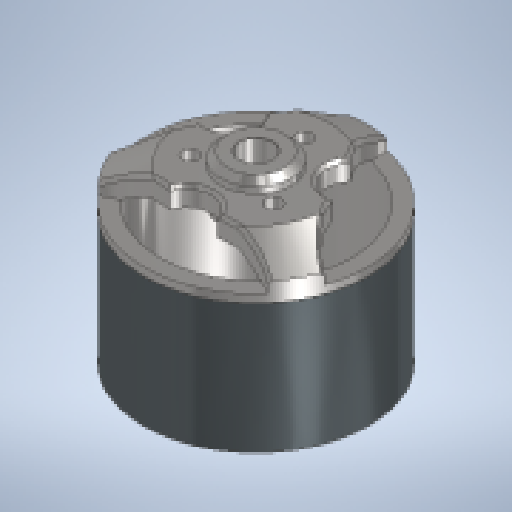
# Autodesk Inventor part: Can
Saved by Autodesk Inventor 2023.2 (Build 272271000, 271)
## iProperties
Created: 2023-03-04
Part Number: Can
Material: Stainless Steel
Document SubType Name: Modeling
Designer: Nathan Cai
Density: 8 g/cm^3
Appearance: Semi-Polished
Author: Nathan Cai
Autodesk Inventor part; units mm, degrees
ref_plane "YZ Plane" through (0, 0, 0) normal (1, 0, 0) x (0, 1, 0)
ref_plane "XZ Plane" through (0, 0, 0) normal (0, 1, 0) x (-1, 0, 0)
ref_plane "XY Plane" through (0, 0, 0) normal (0, 0, 1) x (1, 0, 0)
sketch "Sketch1" plane through (0, 0, 0) normal (0, 1, 0) x (-1, 0, 0)
  line L0 (0, 0) -> (26.5, 0)
  line L1 (26.5, 0) -> (26.5, -17.5)
  line L2 (26.5, -17.5) -> (0, -17.5)
  line L3 (0, -17.5) -> (0, 0)
  line L4 (26.5, -15) -> (0, -15)
  line L5 (0, 0) -> (21.25, 0)
  line L6 (21.25, 0) -> (21.25, -17.5)
  line L7 (21.25, -17.5) -> (0, -17.5)
  line L8 (0, -17.5) -> (0, 0)
  line L9 (26.5, 0) -> (28.5, 0)
  line L10 (28.5, 0) -> (28.5, -5.5)
  line L11 (28.5, -5.5) -> (26.5, -5.5)
  line L12 (26.5, -5.5) -> (26.5, 0)
  line L13 (28.5, 0) -> (0, 0)
  line L14 (0, 0) -> (0, -2.5)
  line L15 (0, -2.5) -> (28.5, -2.5)
  line L16 (28.5, -2.5) -> (28.5, 0)
  line L17 (26.5, -11.5) -> (23.25, -17.5)
  line L18 (26.5, -11.5) -> (23.5, -11.5) construction
  line L19 (23.5, -11.5) -> (23.5, 0)
  line L20 (23.5, 0) -> (26.5, 0)
  line L21 (26.5, 0) -> (26.5, -11.5)
  line L22 (23.5, -11.5) -> (21.6042, -15)
  line L23 (28.5, -5.5) -> (21.25, -5.5)
  line L24 (21.25, -5.5) -> (21.25, 0)
  line L25 (21.25, 0) -> (28.5, 0)
  line L26 (28.5, 0) -> (28.5, -5.5)
  line L27 (0, 0) -> (20.25, 0)
  line L28 (20.25, 0) -> (20.25, -17.55)
  line L29 (20.25, -17.55) -> (0, -17.55)
  line L30 (0, -17.55) -> (0, 0)
  point P0 (28.5, -2.5)
  point P1 (21.25, -2.5)
  point P2 (23.5, -5.5)
  point P3 (20.25, -17.5)
  dimension "d1" = 17.5
  dimension "d2" = 2.5
  dimension "d3" = 21.25
  dimension "d4" = 2
  dimension "d5" = 5.5
  dimension "d6" = 2.5
  dimension "d7" = 11.5
  dimension "d8" = 2
  dimension "d10" = 3
  dimension "d37" = 17.55
  dimension "d38" = 1
  dimension "d39" = 5.25
  constraints: 62 end point, 15 parallel, 8 perpendicular, 8 point on line, 7 horizontal
  measures "d1" distance of L0.end L1.end
  measures "d2" distance between parallel lines of L2 L4
  measures "d3" distance of L6.end L7.end
  measures "d4" distance of L10.end L11.end
  measures "d5" distance of L9.end L10.end
  measures "d6" distance of L14.end L13.end
  measures "d7" distance from line of L13 L17.start
  measures "d8" distance of L17.end L6.end
  measures "d10" distance of L19.end L20.end
  measures "d37" distance of L27.end L28.end
  measures "d38" distance between parallel lines of L6 L28
  measures "d39" distance between parallel lines of L6 L1
revolve "Revolution1" add sketch "Sketch1" angle 360 about axis through (0, 0, 0) along (-1, 0, 0) contours L4 L28 L2 L3 | L15 L19 L23 L6 | L4 L6 L2 L28 | L2 L28 L29 L30 | L15 L1 L23 L19 | L4 L17 L2 L6 | L15 L10 L11 L1 | L23 L1 L17 L4 L22 L19
chamfer "Chamfer1" distance 1 angle 45 1 edges at (-28.5, 0, 5.5)
sketch "Sketch2" plane through (-26.5, 0, 0) normal (-1, 0, 0) x (0, 0, 1)
  circle A0 centre (0, 0) radius 7.5 construction
  line L0 (-7.5, 0) -> (0, 0) construction
  circle A1 centre (-7.5, 0) radius 1.25
  circle A2 centre (0, 0) radius 11 construction
  circle A3 centre (11, 0) radius 4
  circle A4 centre (0, 0) radius 5.5 projected
  circle A5 centre (3.75, -6.4952) radius 1.25
  circle A6 centre (-5.5, 9.5263) radius 4
  circle A7 centre (3.75, 6.4952) radius 1.25
  circle A8 centre (-5.5, -9.5263) radius 4
  point P0 (7, 0)
  point P1 (5.5, 0)
  point P2 (-3.5, 6.0622)
  point P3 (-3.5, -6.0622)
  dimension "d15" = 15
  dimension "d17" = 22
  dimension "d16" = 2.5
  dimension "d19" = 1.5
  dimension "d22" = 360
  constraints: 4 horizontal alignment, 3 centre point, 3 coincident, 3 point on line, 2 end point, 1 horizontal, 29 other
  measures "d16" diameter of A1
  measures "d19" distance of point (5.5, 0) point (7, 0)
extrude "Extrusion1" cut sketch "Sketch2" against normal blind 4 contours A1 | A3 | A5 | A6 | A7 | A8
sketch "Sketch3" plane through (-26.5, 0, 0) normal (-1, 0, 0) x (0, 0, 1)
  line L0 (0, 0) -> (-17.5, 0) construction
  circle A0 centre (0, 0) radius 17.5 projected
  line L1 (-17.1956, 0) -> (-17.1956, 3.25) construction
  arc A1 (-17.1956, 3.25) -> (-3.1605, 17.2122) centre (-17.1956, 17.2852) ccw
  circle A2 centre (-5.5, 9.5263) radius 4 construction
  arc A3 (-8.8511, 7.3422) -> (-1.933, 11.3364) centre (-5.5, 9.5263) ccw projected
  arc A4 (-3.1605, -17.2122) -> (-17.1956, -3.25) centre (-17.1956, -17.2852) ccw
  arc A5 (16.4865, 5.869) -> (11.4124, -13.2668) centre (23.5672, -6.2492) ccw
  arc A6 (5.7832, -16.5168) -> (-13.326, -11.3432) centre (-6.3717, -23.5344) ccw
  arc A7 (-13.326, 11.3432) -> (5.7832, 16.5168) centre (-6.3717, 23.5344) ccw
  arc A8 (11.4124, 13.2668) -> (16.4865, -5.869) centre (23.5672, 6.2492) ccw
  point P0 (-5.5, -9.5263)
  point P1 (11, 0)
  point P2 (-5.5, -9.5263)
  point P3 (-17.1956, -3.25)
  point P4 (5.7832, -16.5168)
  point P5 (-1.5839, 10.3411)
  point P6 (-8.1637, 6.5422)
  point P7 (11, 0)
  point P8 (11.4124, -13.2668)
  point P9 (11.4124, 13.2668)
  dimension "d26" = 3.25
  dimension "d27" = 8
  dimension "d30" = 360
  constraints: 18 point on circle, 7 centre point, 4 end point, 3 symmetric about line, 1 concentric, 1 horizontal, 1 line through centre, 1 point on line, 1 vertical, 30 other
  measures "d26" distance of L1.start L1.end
  measures "d27" diameter of A2
extrude "Extrusion2" cut sketch "Sketch3" against normal blind 5 contours A0 A8 A5 | A5 A8 A0 | A0 A5 A8 | A7 A1 A0 | A0 A4 A6 | A1 A7 A0 | A3 A1 A7 | A0 A6 A4 | A6 A0 A4 | A7 A1 A0
chamfer "Chamfer2" distance 0.5 angle 45 15 edges at (-24.9582, -10.1916, 10.0971) (-26.5, -5.1103, 9.5783) (-26.5, 0, 7) (-26.5, 5.1103, 9.5783) (-24.9582, 10.1916, 10.0971) (-24.9582, 13.8401, 3.7776) (-26.5, 10.8502, -0.3635) (-26.5, 6.0622, -3.5) (-26.5, 5.7399, -9.2148) (-24.9582, 3.6485, -13.8748) (-24.9582, -3.6485, -13.8747) (-26.5, -5.7399, -9.2148) (-26.5, -6.0622, -3.5) (-26.5, -10.8502, -0.3635) (-24.9582, -13.8401, 3.7777)
chamfer "Chamfer3" distance 0.1 angle 45 1 edges at (-28.5, 0, 2.5)
body "Solid1"
